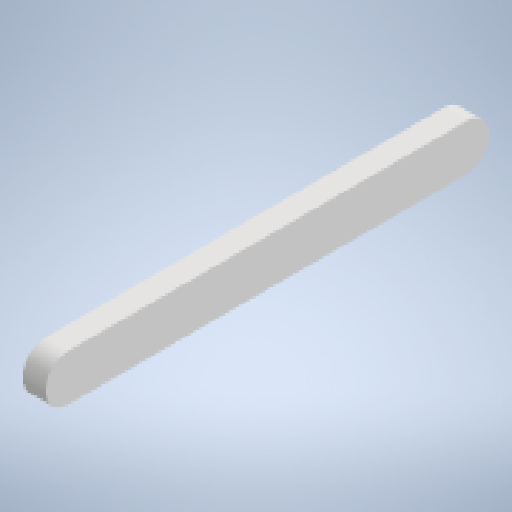
# Autodesk Inventor part: Link A
Saved by Autodesk Inventor 2023 (Build 270158000, 158)
## iProperties
Created: 2024-01-19
Part Number: Link A
Material: Generic
Document SubType Name: Modeling
Designer: juanp
Density: 1 g/cm^3
Appearance: Default
Author: juanp
Autodesk Inventor part; units mm, degrees
ref_plane "YZ Plane" through (0, 0, 0) normal (1, 0, 0) x (0, 1, 0)
ref_plane "XZ Plane" through (0, 0, 0) normal (0, 1, 0) x (-1, 0, 0)
ref_plane "XY Plane" through (0, 0, 0) normal (0, 0, 1) x (1, 0, 0)
sketch "Sketch1" plane through (0, 0, 0) normal (1, 0, 0) x (0, 1, 0)
  line L0 (0, -43) -> (0, 43) construction
  line L1 (5, -43) -> (5, 43)
  line L2 (-5, 43) -> (-5, -43)
  arc A0 (-5, -43) -> (5, -43) centre (0, -43) ccw
  arc A1 (5, 43) -> (-5, 43) centre (0, 43) ccw
  point P0 (0, 0)
  dimension "d0" = 86
  dimension "d5" = 10
  constraints: 8 end point, 4 point on circle, 4 tangent, 2 centre point, 1 midpoint, 1 parallel, 1 vertical
  measures "d0" distance of L0.start L0.end
  measures "d5" distance between parallel lines of L1 L2
extrude "Extrusion1" add sketch "Sketch1" along normal blind 10
body "Solid1"
